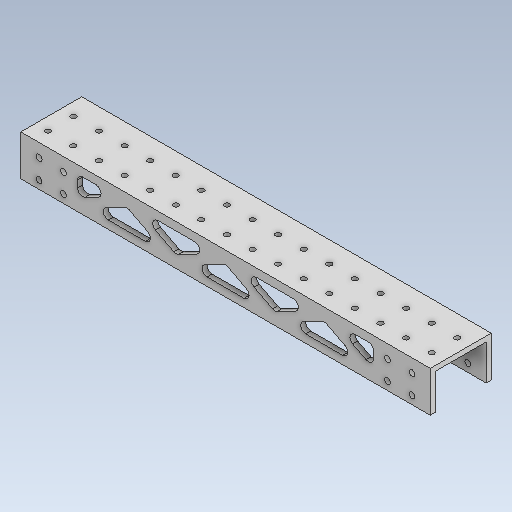
# Autodesk Inventor part: middleBar
Saved by Autodesk Inventor 2021 (Build 250183000, 183)
## iProperties
Created: 2020-03-21
Part Number: middleBar
Material: Generic
Document SubType Name: Modeling
Designer: deli
Density: 1 g/cm^3
Appearance: Default
Author: deli
Autodesk Inventor part; units mm, degrees
ref_plane "YZ Plane" through (0, 0, 0) normal (1, 0, 0) x (0, 1, 0)
ref_plane "XZ Plane" through (0, 0, 0) normal (0, 1, 0) x (-1, 0, 0)
ref_plane "XY Plane" through (0, 0, 0) normal (0, 0, 1) x (1, 0, 0)
sketch "Sketch1" plane through (0, 0, 0) normal (1, 0, 0) x (0, 1, 0)
  line L0 (24.8759, -34.1824) -> (21.7009, -34.1824)
  line L1 (21.7009, -34.1824) -> (21.7009, -72.2824)
  line L2 (21.7009, -72.2824) -> (24.8759, -72.2824)
  line L3 (24.8759, -72.2824) -> (24.8759, -34.1824)
  line L4 (24.8759, -34.1824) -> (-0.5241, -34.1824)
  line L5 (-0.5241, -34.1824) -> (-0.5241, -37.3574)
  line L6 (-0.5241, -37.3574) -> (24.8759, -37.3574)
  line L7 (24.8759, -37.3574) -> (24.8759, -34.1824)
  line L8 (24.8759, -72.2824) -> (-0.5241, -72.2824)
  line L9 (-0.5241, -72.2824) -> (-0.5241, -69.1074)
  line L10 (-0.5241, -69.1074) -> (24.8759, -69.1074)
  line L11 (24.8759, -69.1074) -> (24.8759, -72.2824)
  point P0 (0, 0)
  point P1 (21.7009, -37.3574)
  point P2 (21.7009, -69.1074)
  dimension "d0" = 3.175
  dimension "d1" = 38.1
  dimension "d2" = 25.4
  dimension "d3" = 3.175
  dimension "d4" = 3.175
  dimension "d5" = 25.4
  constraints: 24 end point, 6 parallel, 3 horizontal, 3 perpendicular
  measures "d0" distance of L2.end L1.end
  measures "d1" distance of L1.end L0.end
  measures "d2" distance of L6.end L5.end
  measures "d3" distance of L5.end L4.end
  measures "d4" distance of L8.end L9.end
  measures "d5" distance of L9.end L10.end
extrude "Extrusion1" add sketch "Sketch1" along normal blind 256.0026
sketch "Sketch2" plane through (0, -0.5241, -34.1824) normal (0, 0, 1) x (1, 0, 0)
  circle A0 centre (11.43, 17.145) radius 1.8542 projected
  circle A1 centre (11.43, 5.08) radius 1.8542 projected
  circle A2 centre (26.67, 5.08) radius 1.8542 projected
  circle A3 centre (26.67, 17.145) radius 1.8542 projected
  circle A4 centre (244.5726, 5.08) radius 1.8542 projected
  circle A5 centre (229.3326, 5.08) radius 1.8542 projected
  circle A6 centre (229.3326, 17.145) radius 1.8542 projected
  circle A7 centre (244.5726, 17.145) radius 1.8542 projected
  point P0 (0, 0.5241)
extrude "Extrusion2" cut sketch "Sketch2" against normal blind 76.2
sketch "Sketch3" plane through (0, 24.8759, -34.1824) normal (0, 1, 0) x (1, 0, 0)
  circle A0 centre (8, 24.9) radius 1.65
  line L0 (0, 38.1) -> (0, 0) projected
  line L1 (0, 0) -> (256.0026, 0) projected
  line L2 (256.0026, 38.1) -> (256.0026, 0) projected
  line L3 (0, 38.1) -> (256.0026, 38.1) projected
  circle A1 centre (8, 8.9) radius 1.65
  circle A2 centre (24, 24.9) radius 1.65
  circle A3 centre (24, 8.9) radius 1.65
  circle A4 centre (40, 24.9) radius 1.65
  circle A5 centre (40, 8.9) radius 1.65
  circle A6 centre (56, 24.9) radius 1.65
  circle A7 centre (56, 8.9) radius 1.65
  circle A8 centre (72, 24.9) radius 1.65
  circle A9 centre (72, 8.9) radius 1.65
  circle A10 centre (88, 24.9) radius 1.65
  circle A11 centre (88, 8.9) radius 1.65
  circle A12 centre (104, 24.9) radius 1.65
  circle A13 centre (104, 8.9) radius 1.65
  circle A14 centre (120, 24.9) radius 1.65
  circle A15 centre (120, 8.9) radius 1.65
  circle A16 centre (136, 24.9) radius 1.65
  circle A17 centre (136, 8.9) radius 1.65
  circle A18 centre (151.9999, 24.9) radius 1.65
  circle A19 centre (151.9999, 8.9) radius 1.65
  circle A20 centre (167.9999, 24.9) radius 1.65
  circle A21 centre (167.9999, 8.9) radius 1.65
  circle A22 centre (183.9999, 24.9) radius 1.65
  circle A23 centre (183.9999, 8.9) radius 1.65
  circle A24 centre (199.9999, 24.9) radius 1.65
  circle A25 centre (199.9999, 8.9) radius 1.65
  circle A26 centre (215.9999, 24.9) radius 1.65
  circle A27 centre (215.9999, 8.9) radius 1.65
  line L4 (223.9999, 29.6543) -> (223.9999, 8.188)
  circle A28 centre (-8, 40.9) radius 1.65 projected
  circle A29 centre (-8, 24.9) radius 1.65 projected
  circle A30 centre (231.9999, 24.9) radius 1.65
  circle A31 centre (247.9999, 24.9) radius 1.65
  circle A32 centre (215.9999, 8.9) radius 1.65
  circle A33 centre (231.9999, 8.9) radius 1.65
  circle A34 centre (247.9999, 8.9) radius 1.65
  point P0 (0, -34.1824)
  dimension "d10" = 3.3
  dimension "d13" = 16
  dimension "d16" = 16
  dimension "d19" = 8
  dimension "d20" = 8
  dimension "d21" = 223.9999
  dimension "d26" = 16
  dimension "d29" = 16
  dimension "d32" = 0
  constraints: 33 centre point, 3 vertical, 2 end point, 2 horizontal, 64 other
  measures "d10" diameter of A0
  measures "d13" distance of A0.centre A1.centre
  measures "d16" distance of A0.centre A2.centre
  measures "d19" distance from line of A1.centre L0
  measures "d20" distance from line of L4 A26.centre
  measures "d21" distance between parallel lines of L4 L0
  measures "d26" distance of A26.centre A30.centre
  measures "d29" distance of A26.centre A32.centre
  measures "d32" vertical distance of A0.centre A29.centre
extrude "Extrusion3" cut sketch "Sketch3" against normal blind 25.4 contours A0 | A1 | A2 | A3 | A4 | A5 | A6 | A7 | A8 | A9 | A10 | A11 | A12 | A13 | A14 | A15 | A16 | A17 | A18 | A19 | A20 | A21 | A22 | A23 | A24 | A25 | A26 | A27 | A30 | A31 | A33 | A34
sketch "Sketch4" plane through (0, -0.5241, -34.1824) normal (0, 0, 1) x (1, 0, 0)
  circle A0 centre (26.67, 17.145) radius 1.8542 projected
  circle A1 centre (229.3326, 5.08) radius 1.8542 projected
  circle A2 centre (244.5726, 17.145) radius 1.8542 projected
  circle A3 centre (11.43, 5.08) radius 1.8542 projected
  circle A4 centre (26.67, 5.08) radius 1.8542 projected
  circle A5 centre (244.5726, 5.08) radius 1.8542 projected
  circle A6 centre (229.3326, 17.145) radius 1.8542 projected
  circle A7 centre (11.43, 17.145) radius 1.8542 projected
  line L0 (0, 25.4) -> (0, 0) projected
  line L1 (0, 0) -> (256.0026, 0) projected
  line L2 (256.0026, 25.4) -> (256.0026, 0) projected
  line L3 (0, 25.4) -> (256.0026, 25.4) projected
  line L4 (250.9226, 20.32) -> (250.9226, 5.08)
  line L5 (250.9226, 5.08) -> (5.08, 5.08)
  line L6 (5.08, 5.08) -> (5.08, 20.32)
  line L7 (5.08, 20.32) -> (250.9226, 20.32)
  line L8 (35.4584, 20.32) -> (35.4584, 5.08)
  line L9 (220.5442, 20.32) -> (220.5442, 5.08)
  line L10 (35.4584, 5.08) -> (64.932, 5.08)
  line L11 (41.6249, 5.08) -> (66.306, 17.78)
  line L12 (60.1395, 20.32) -> (86.2983, 20.32)
  line L13 (66.306, 17.78) -> (90.9871, 5.08)
  line L14 (103.3202, 5.08) -> (128.0013, 17.78)
  line L15 (103.3202, 5.08) -> (109.434, 5.08)
  line L16 (134.1678, 20.32) -> (158.8489, 7.62)
  line L17 (134.1678, 20.32) -> (132.5697, 20.32)
  line L18 (165.0155, 5.08) -> (189.6966, 17.78)
  line L19 (165.0155, 5.08) -> (155.7054, 5.08)
  line L20 (97.1537, 7.62) -> (121.8347, 20.32)
  line L21 (128.0013, 17.78) -> (152.6824, 5.08)
  line L22 (183.53, 20.32) -> (158.8489, 7.62)
  line L23 (97.1537, 7.62) -> (72.4726, 20.32)
  line L24 (189.6966, 17.78) -> (214.3776, 5.08)
  line L25 (60.1395, 20.32) -> (35.4584, 7.62)
  line L26 (195.8631, 20.32) -> (220.5442, 7.62)
  point P0 (0, 0.5241)
  point P1 (156.3402, 20.32)
  point P2 (179.4759, 5.08)
  point P3 (202.2924, 20.32)
  point P4 (169.0696, 5.08)
  point P5 (192.2053, 20.32)
  point P6 (212.6183, 5.08)
  point P7 (165.0155, 5.08)
  point P8 (195.3165, 20.32)
  dimension "d33" = 5.08
  dimension "d34" = 8.7884
  dimension "d35" = 3.7084
  dimension "d36" = 8.7884
  dimension "d52" = 185.0858
  dimension "d59" = 5.08
  dimension "d60" = 5.08
  dimension "d64" = 61.6953
  dimension "d66" = 12.7
  dimension "d67" = 5.08
  dimension "d68" = 12.7
  dimension "d69" = 12.7
  dimension "d70" = 12.7
  dimension "d73" = 12.7
  dimension "d74" = 30.8476
  dimension "d75" = 5.08
  dimension "d80" = 61.6953
  dimension "d82" = 61.6953
  dimension "d83" = 61.6953
  dimension "d88" = 12.7
  dimension "d89" = 5.08
  dimension "d90" = 5.08
  dimension "d91" = 12.7
  constraints: 42 end point, 6 parallel, 5 horizontal, 4 point on line, 2 vertical, 30 other
  measures "d34" distance from line of L8 A0.centre
  measures "d35" diameter of A0
  measures "d36" distance from line of A6.centre L9
  measures "d52" distance between parallel lines of L9 L8
  measures "d59" distance between parallel lines of L14 L20
  measures "d60" distance between parallel lines of L18 L22
  measures "d64" horizontal distance of L20.start L8.end
  measures "d67" distance between parallel lines of L16 L21
  measures "d69" distance from line of L14.end L15
  measures "d74" horizontal distance of L8.end L11.end
  measures "d75" distance between parallel lines of L23 L13
  measures "d80" distance of L20.start L16.end
  measures "d82" distance of L14.end L11.end
  measures "d83" distance of L18.end L14.end
  measures "d89" distance between parallel lines of L26 L24
  measures "d90" distance between parallel lines of L11 L25
extrude "Extrusion4" cut sketch "Sketch4" against normal blind 76.2 contours L5 L18 L24 | L26 L7 L9 | L22 L16 L7 | L5 L14 L21 | L20 L23 L7 | L5 L11 L13 | L25 L8 L7
fillet "Fillet2" radius 3.175 42 edges at (35.4584, 19.7959, -35.7699) (60.1395, 19.7959, -70.6949) (60.1395, 19.7959, -35.7699) (66.306, 17.2559, -35.7699) (41.6249, 4.5559, -35.7699) (90.9871, 4.5559, -35.7699) (97.1537, 7.0959, -35.7699) (72.4726, 19.7959, -35.7699) (121.8347, 19.7959, -35.7699) (103.3202, 4.5559, -35.7699) (128.0013, 17.2559, -35.7699) (152.6824, 4.5559, -35.7699) (134.1678, 19.7959, -35.7699) (183.53, 19.7959, -35.7699) (158.8489, 7.0959, -35.7699) (165.0155, 4.5559, -35.7699) (189.6966, 17.2559, -35.7699) (214.3776, 4.5559, -35.7699) (220.5442, 19.7959, -35.7699) (220.5442, 19.7959, -70.6949) (189.6966, 17.2559, -70.6949) (214.3776, 4.5559, -70.6949) (165.0155, 4.5559, -70.6949) (183.53, 19.7959, -70.6949) (158.8489, 7.0959, -70.6949) (152.6824, 4.5559, -70.6949) (134.1678, 19.7959, -70.6949) (128.0013, 17.2559, -70.6949) (103.3202, 4.5559, -70.6949) (97.1537, 7.0959, -70.6949) (90.9871, 4.5559, -70.6949) (41.6249, 4.5559, -70.6949) (35.4584, 19.7959, -70.6949) (72.4726, 19.7959, -70.6949) (121.8347, 19.7959, -70.6949) (66.306, 17.2559, -70.6949) (35.4584, 7.0959, -35.7699) (195.8631, 19.7959, -35.7699) (220.5442, 7.0959, -35.7699) (220.5442, 7.0959, -70.6949) (195.8631, 19.7959, -70.6949) (35.4584, 7.0959, -70.6949)
equation "\"d4\" = d3"
equation "\"d5\" = d2"
equation "\"d36\" = d34"
equation "\"d59\" = d38"
equation "\"d60\" = d38"
equation "\"d67\" = d59"
equation "\"d74\" = 0.5 * d64"
equation "\"d75\" = d38"
equation "\"d38\" = 5.08"
body "Solid1"
